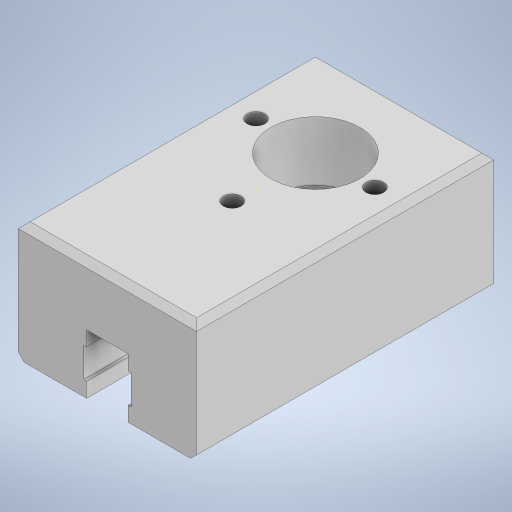
# Autodesk Inventor part: Schneidführung
Saved by Autodesk Inventor 2023.2 (Build 272271030, 271C)
## iProperties
Created: 2023-02-12
Part Number: Schneidführung
Material: Generic
Document SubType Name: Modeling
Designer: Ayush
Density: 1 g/cm^3
Appearance: Default
Author: Ayush
Autodesk Inventor part; units mm, degrees
ref_plane "YZ Plane" through (0, 0, 0) normal (1, 0, 0) x (0, 1, 0)
ref_plane "XZ Plane" through (0, 0, 0) normal (0, 1, 0) x (-1, 0, 0)
ref_plane "XY Plane" through (0, 0, 0) normal (0, 0, 1) x (1, 0, 0)
sketch "Sketch1" plane through (0, 0, 0) normal (0, 1, 0) x (-1, 0, 0)
  line L0 (-30, 50) -> (30, 50)
  line L1 (30, 50) -> (30, -50)
  line L2 (30, -50) -> (-30, -50)
  line L3 (-30, -50) -> (-30, 50)
  line L4 (-30, 50) -> (30, -50) construction
  line L5 (30, 50) -> (-30, -50) construction
  circle A0 centre (0, 8) radius 3
  circle A1 centre (20, -20) radius 3
  circle A2 centre (-20, -20) radius 3
  circle A3 centre (0, -20) radius 15
  point P0 (0, 0)
  dimension "d0" = 60
  dimension "d1" = 100
  dimension "d2" = 6
  dimension "d3" = 6
  dimension "d5" = 58
  dimension "d6" = 10
  dimension "d8" = 30
  dimension "d9" = 6
  dimension "d10" = 10
  dimension "d11" = 30
  dimension "d12" = 30
  constraints: 12 end point, 4 centre point, 2 midpoint, 2 parallel, 2 vertical alignment, 1 horizontal, 1 horizontal alignment, 1 perpendicular
  measures "d0" distance of L1.end L2.end
  measures "d1" distance of L0.end L1.end
  measures "d2" diameter of A0
  measures "d3" diameter of A1
  measures "d5" distance from line of A0.centre L2
  measures "d6" distance from line of L1 A1.centre
  measures "d8" distance from line of A1.centre L2
  measures "d9" diameter of A2
  measures "d10" distance from line of A2.centre L3
  measures "d11" diameter of A3
  measures "d12" distance from line of A3.centre L2
extrude "Extrusion1" add sketch "Sketch1" along normal blind 20
sketch "Sketch2" plane through (0, 0, 0) normal (0, -1, 0) x (1, 0, 0)
  line L0 (30, -50) -> (-30, -50) projected
  line L1 (7, -50) -> (7, 50)
  line L2 (-7, -50) -> (-7, 50)
  line L3 (30, 50) -> (30, -50) projected
  line L4 (-30, -50) -> (-30, 50) projected
  line L5 (7, -50) -> (30, -50)
  line L6 (30, 50) -> (30, -50) projected
  line L7 (30, 50) -> (7, 50)
  line L8 (-30, 50) -> (30, 50) projected
  line L9 (-7, -50) -> (-30, -50)
  line L10 (-30, -50) -> (-30, 50) projected
  line L11 (-30, 50) -> (-7, 50)
  point P0 (0, 0)
  dimension "d15" = 23
  dimension "d16" = 23
  constraints: 12 end point, 3 collinear, 2 point on line, 2 vertical, 1 parallel
  measures "d15" distance between parallel lines of L1 L3
  measures "d16" distance between parallel lines of L2 L4
extrude "Extrusion2" add sketch "Sketch2" along normal blind 5 contours L0 L1 L7 L3 | L0 L4 L8 L2
sketch "Sketch3" plane through (0, -5, 0) normal (0, -1, 0) x (1, 0, 0)
  line L0 (30, -50) -> (-30, -50) projected
  line L1 (8, -50) -> (8, 50)
  line L2 (-30, 50) -> (30, 50) projected
  line L3 (-8, -50) -> (-8, 50)
  line L4 (30, -50) -> (30, 50) projected
  line L5 (-30, 50) -> (-30, -50) projected
  line L6 (8, -50) -> (30, -50)
  line L7 (30, 50) -> (30, -50) projected
  line L8 (30, 50) -> (8, 50)
  line L9 (-8, 50) -> (-30, 50)
  line L10 (-30, -50) -> (-8, -50)
  point P0 (0, 0)
  dimension "d19" = 22
  dimension "d20" = 22
  constraints: 12 end point, 4 point on line, 3 collinear, 2 vertical, 1 perpendicular
  measures "d19" distance between parallel lines of L1 L4
  measures "d20" distance between parallel lines of L5 L3
extrude "Extrusion3" add sketch "Sketch3" along normal blind 10 contours L0 L1 L2 L4 | L0 L5 L2 L3
sketch "Sketch4" plane through (0, -15, 0) normal (0, -1, 0) x (1, 0, 0)
  line L0 (8, -50) -> (30, -50) projected
  line L1 (7, -50) -> (7, 50)
  line L2 (-30, 50) -> (30, 50) projected
  line L3 (-30, -50) -> (-8, -50) projected
  line L4 (30, -50) -> (30, 50) projected
  line L5 (-30, 50) -> (-30, -50) projected
  line L6 (7, -50) -> (30, -50)
  line L7 (30, 50) -> (30, -50) projected
  line L8 (30, 50) -> (7, 50)
  line L9 (-30, -50) -> (-30, 50) projected
  line L10 (-30, -50) -> (-30, 50)
  line L11 (-30, -50) -> (-7, -50)
  line L12 (-30, 50) -> (-7, 50)
  line L13 (-7, 50) -> (-7, -50)
  point P0 (0, 0)
  dimension "d23" = 23
  dimension "d25" = 23
  dimension "d26" = 100
  constraints: 14 end point, 4 point on line, 3 collinear, 1 vertical
  measures "d23" distance between parallel lines of L1 L4
  measures "d25" distance of L3.start L11.end
  measures "d26" distance of L12.end L11.end
extrude "Extrusion4" add sketch "Sketch4" along normal blind 5
sketch "Sketch5" plane through (0, -20, 0) normal (0, -1, 0) x (1, 0, 0)
  circle A0 centre (17, -35) radius 3
  circle A1 centre (17, 0) radius 3
  circle A2 centre (17, 35) radius 3
  circle A3 centre (-17, 35) radius 3
  circle A4 centre (-17, 0) radius 3
  circle A5 centre (-17, -35) radius 3
  line L0 (-7, 50) -> (-30, 50) projected
  line L1 (-30, 50) -> (-30, -50) projected
  line L2 (30, -50) -> (30, 50) projected
  point P0 (0, 0)
  dimension "d29" = 6
  dimension "d30" = 6
  dimension "d31" = 6
  dimension "d32" = 6
  dimension "d33" = 6
  dimension "d34" = 6
  dimension "d35" = 15
  dimension "d36" = 35
  dimension "d37" = 70
  dimension "d38" = 13
  dimension "d39" = 13
  constraints: 6 centre point, 4 vertical alignment, 3 horizontal alignment
  measures "d29" diameter of A0
  measures "d30" diameter of A1
  measures "d31" diameter of A2
  measures "d32" diameter of A3
  measures "d33" diameter of A4
  measures "d34" diameter of A5
  measures "d35" distance from line of A3.centre L0
  measures "d36" distance of A4.centre A3.centre
  measures "d37" distance of A5.centre A3.centre
  measures "d38" distance from line of A3.centre L1
  measures "d39" distance from line of L2 A2.centre
hole "Hole1" at (17, -20, -35) at (17, -20, 0) at (17, -20, 35) at (-17, -20, 35) at (-17, -20, 0) at (-17, -20, -35) direction (0, 1, 0) diameter 6 depth 9 tip angle 118
chamfer "Chamfer1" distance 2 angle 45 1 edges at (30, -20, 0) measured on face at (26.6594, -20, 0.1205)
chamfer "Chamfer2" distance 2 angle 45 1 edges at (-30, -20, 0) measured on face at (-26.6594, -20, -0.1205)
chamfer "Chamfer3" distance 2 angle 45 1 edges at (30, 20, 0) measured on face at (0.1205, 20, 36.9927)
chamfer "Chamfer4" distance 2 angle 45 1 edges at (-30, 20, 0) measured on face at (-0.7872, 20, 36.9927)
chamfer "Chamfer5" distance 2 angle 45 1 edges at (0, 20, -50) measured on face at (-0.1205, 20, 36.9927)
chamfer "Chamfer6" distance 2 angle 45 1 edges at (0, 20, 50) measured on face at (0.1205, 20, 36.9927)
sketch "Sketch6" plane through (7, 0, -50) normal (0, 0, -1) x (-1, 0, 0)
  circle A0 centre (17, 10) radius 4
  circle A1 centre (-3, 10) radius 4
  line L0 (37, -18) -> (37, 18) projected
  line L1 (-23, 18) -> (-23, -18) projected
  line L2 (35, 20) -> (-21, 20) projected
  point P0 (7, 0)
  dimension "d65" = 8
  dimension "d66" = 8
  dimension "d67" = 20
  dimension "d68" = 20
  dimension "d69" = 10
  constraints: 2 centre point, 1 horizontal alignment
  measures "d65" diameter of A0
  measures "d66" diameter of A1
  measures "d67" distance from line of A0.centre L0
  measures "d68" distance from line of A1.centre L1
  measures "d69" distance from line of A1.centre L2
hole "Hole2" at (10, 10, -50) at (-10, 10, -50) direction (0, 0, 1) diameter 8 depth 12 tip angle 118
sketch "Sketch7" plane through (0, 20, 0) normal (0, 1, 0) x (1, 0, 0)
  point P0 (0, 0)
sketch "Sketch8" plane through (0, 0, 0) normal (0, -1, 0) x (1, 0, 0)
  line L0 (6.6295, 50) -> (7, 0)
  line L1 (7, -6.7335) -> (7, 50) projected
  line L2 (-7, 50) -> (-7, -6.7335) projected
  line L3 (-7, 0) -> (-7, 50)
  line L4 (-7, 50) -> (6.6295, 50)
  line L5 (-7, 50) -> (7, 50) projected
  line L6 (7, 0) -> (-7, 0)
  point P0 (0, 0)
  constraints: 8 end point, 2 collinear, 2 point on line, 1 horizontal
extrude "Extrusion5" add sketch "Sketch8" along normal blind 0.01 contours L0 L6 L2 L4
sketch "Sketch9" plane through (0, 20, 0) normal (0, 1, 0) x (1, 0, 0)
  circle A0 centre (0, -8) radius 3
  line L0 (30, 50) -> (-30, 50) projected
  point P0 (0, 0)
  dimension "d79" = 6
  dimension "d80" = 58
  constraints: 1 centre point
  measures "d79" diameter of A0
  measures "d80" distance from line of A0.centre L0
hole "Hole3" at (0, 20, 8) direction (0, -1, 0) diameter 6 depth 10 tip angle 118
body "Solid1"
